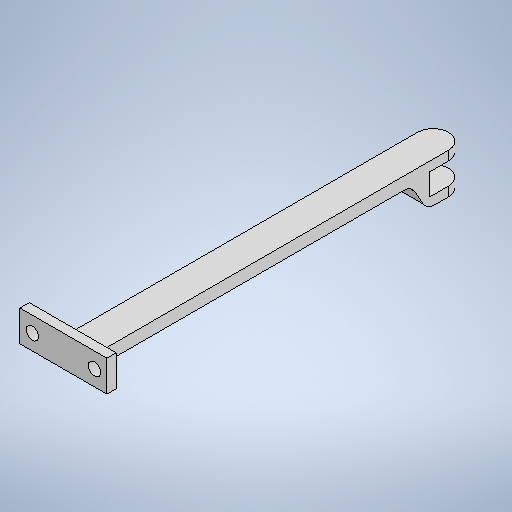
# Autodesk Inventor part: 2052
Saved by Autodesk Inventor 2025 (Build 290162010, 162A)
## iProperties
Created: 2024-06-01
Part Number: 2052
Material: Generic
Document SubType Name: Modeling
Designer: Fabri
Density: 1 g/cm^3
Appearance: Default
Author: Fabri
Autodesk Inventor part; units mm, degrees
ref_plane "YZ Plane" through (0, 0, 0) normal (1, 0, 0) x (0, 1, 0)
ref_plane "XZ Plane" through (0, 0, 0) normal (0, 1, 0) x (-1, 0, 0)
sketch "Sketch5" plane through (0, 0, 0) normal (1, 0, 0) x (0, 1, 0)
  line L0 (0, 0) -> (98.4806, 0)
  line L1 (98.4806, 0) -> (98.4806, -3)
  line L2 (98.4806, -3) -> (87.4806, -3)
  line L3 (87.4806, -3) -> (87.4806, -10)
  line L4 (87.4806, -10) -> (98.4806, -10)
  line L5 (98.4806, -10) -> (98.4806, -13)
  line L6 (98.4806, -13) -> (86.4806, -13)
  line L7 (86.4806, -13) -> (81.4806, -4)
  line L8 (-22.5194, 0) -> (0, 0)
  line L9 (-22.5194, -4) -> (81.4806, -4)
  line L10 (-22.5194, -4) -> (-22.5194, 0)
  dimension "d29" = 3
  dimension "d30" = 7
  dimension "d31" = 3
  dimension "d33" = 11
  dimension "d40" = 4
  dimension "d41" = 5
  dimension "d48" = 12
  dimension "d53" = 121
  constraints: 22 end point, 5 perpendicular, 2 horizontal, 2 point on line, 1 vertical
  measures "d29" distance between parallel lines of L2 L0
  measures "d30" distance between parallel lines of L4 L2
  measures "d31" distance between parallel lines of L6 L4
  measures "d33" distance between parallel lines of L3 L1
  measures "d40" distance between parallel lines of L9 L8
  measures "d41" horizontal distance of L6.end L7.end
  measures "d48" distance of L5.end L6.end
  measures "d53" distance from line of L1.end L10
ref_plane "Work Plane1" through (0, 0, 0) normal (0, 0, 1) x (1, 0, 0)
extrude "Extrusion5" add sketch "Sketch5" along normal blind 10
fillet "Fillet1" radius 5 4 edges at (10, 98.4806, -11.5) (0, 98.4806, -11.5) (0, 98.4806, -1.5) (10, 98.4806, -1.5)
fillet "Fillet2" radius 4 2 edges at (5, 86.4806, -13) (5, 81.4806, -4)
sketch "Sketch7" plane through (0, -22.5194, -4) normal (0, 0, -1) x (1, 0, 0)
  line L0 (-9, 0) -> (19, 0)
  line L1 (19, 0) -> (19, 3)
  line L2 (19, 3) -> (-9, 3)
  line L3 (-9, 3) -> (-9, 0)
  line L4 (10, -107.857) -> (0, -107.857) projected
  line L5 (10, -101.6464) -> (0, -101.6464) projected
  line L6 (10, 0) -> (10, -101.6464) projected
  line L7 (0, 0) -> (10, 0) projected
  line L8 (0, 0) -> (0, -101.6464) projected
  point P0 (5, 3)
  point P1 (5, -107.857)
  point P2 (5, 0)
  dimension "d58" = 28
  dimension "d59" = 3
  constraints: 8 end point, 4 midpoint, 2 parallel, 1 horizontal, 1 perpendicular, 1 other
  measures "d58" distance between parallel lines of L3 L1
  measures "d59" distance between parallel lines of L0 L2
extrude "Extrusion6" add sketch "Sketch7" against normal blind 10 contours L3 L2 L1 L0
sketch "Sketch8" plane through (-9, -22.5194, -4) normal (0, 1, 0) x (1, 0, 0)
  line L0 (0, 0) -> (0, -10) projected
  line L1 (28, 0) -> (28, -10) projected
  point P0 (9, -4)
  point P1 (4, -5)
  point P2 (24, -5)
  point P3 (0, -5)
  point P4 (28, -5)
  dimension "d69" = 4
  dimension "d70" = 4
  constraints: 2 horizontal alignment, 2 midpoint
  measures "d69" distance from line of point (4, -5) L0
  measures "d70" distance from line of L1 point (24, -5)
hole "Hole3" at (-5, -22.5194, 1) at (15, -22.5194, 1) direction (0, -1, 0) diameter 4 end through all
equation "\"d31\" = d29"
body "Solid3"
